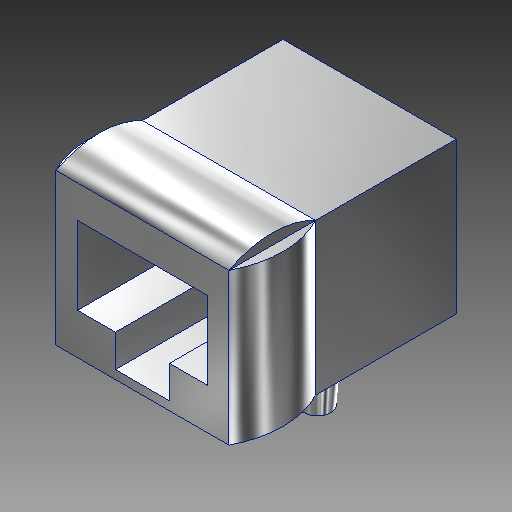
# Autodesk Inventor part: RJ45 Socket
Saved by Autodesk Inventor 2019.4 (Build 234330000, 330)
## iProperties
Created: 2014-11-01
Part Number: RJ45 Socket
Material: Aluminium 6061
Document SubType Name: Modeling
Designer: AndreR
Mass: 10.7449 g
Surface Area: 22.49 cm^2
Volume: 3.96489 cm^3
Density: 2.71 g/cm^3
Appearance: Aluminium - flach
Author: AndreR
Autodesk Inventor part; units mm, degrees
ref_plane "YZ Plane" through (0, 0, 0) normal (1, 0, 0) x (0, 1, 0)
ref_plane "XZ Plane" through (0, 0, 0) normal (0, 1, 0) x (-1, 0, 0)
ref_plane "XY Plane" through (0, 0, 0) normal (0, 0, 1) x (1, 0, 0)
sketch "Skizze1" plane through (0, 0, 0) normal (0, 0, 1) x (1, 0, 0)
  line L0 (-8, 10.5) -> (8, 10.5)
  line L1 (8, 10.5) -> (8, -10.5)
  line L2 (8, -10.5) -> (-8, -10.5)
  line L3 (-8, -10.5) -> (-8, 10.5)
  line L4 (0, 14.7) -> (0, -14.7) projected
  line L5 (-11.2, 0) -> (11.2, 0) projected
  point P0 (0, 0)
  dimension "d0" = 16
  dimension "d2" = 21
  constraints: 8 end point, 2 parallel, 1 horizontal, 1 perpendicular, 2 other
  measures "d0" distance of L0.start L0.end
  measures "d2" distance of L2.end L0.start
extrude "Extrusion1" add sketch "Skizze1" along normal blind 14
sketch "Skizze2" plane through (-8, -10.5, 0) normal (0, -1, 0) x (1, 0, 0)
  line L0 (2, 11) -> (14, 11)
  line L1 (14, 11) -> (14, 3.8)
  line L2 (2, 3.8) -> (2, 11)
  line L3 (10.5, 3.8) -> (10.5, 0.8)
  line L4 (10.5, 0.8) -> (5.5, 0.8)
  line L5 (5.5, 0.8) -> (5.5, 3.8)
  line L6 (16, 0) -> (0, 0) projected
  line L7 (16, 0) -> (16, 14) projected
  line L8 (0, 14) -> (16, 14) projected
  line L9 (0, 0) -> (0, 14) projected
  line L10 (8, 14) -> (8, 0) construction
  line L11 (14, 3.8) -> (10.5, 3.8)
  line L12 (5.5, 3.8) -> (2, 3.8)
  dimension "d5" = 3
  dimension "d6" = 0.8
  dimension "d8" = 2
  dimension "d9" = 5
  dimension "d10" = 3
  constraints: 18 end point, 4 parallel, 2 perpendicular, 1 horizontal, 1 midpoint, 3 other
  measures "d5" distance between parallel lines of L0 L8
  measures "d6" distance between parallel lines of L4 L6
  measures "d8" distance between parallel lines of L1 L7
  measures "d9" distance of L3.end L4.end
  measures "d10" distance between parallel lines of L4 L11
extrude "Extrusion2" cut sketch "Skizze2" against normal blind 10 contours L0 L1 L11 L3 L4 L5 L12 L2
sketch "Skizze3" plane through (0, 0, 0) normal (0, 0, -1) x (-1, 0, 0)
  line L0 (-8, -10.5) -> (8, -10.5) projected
  line L1 (-8, 10.5) -> (-8, -10.5) projected
  line L2 (8, -10.5) -> (8, 10.5) projected
  line L3 (-5.7, 0) -> (5.7, 0) construction
  line L4 (0, -14.7) -> (0, 14.7) construction
  circle A0 centre (-5.7, 0) radius 1.5
  circle A1 centre (5.7, 0) radius 1.5
  point P0 (0, 0)
  dimension "d13" = 10.5
  dimension "d14" = 11.4
  dimension "d15" = 3
  dimension "d16" = 3
  constraints: 2 centre point, 2 coincident, 2 end point, 1 perpendicular, 1 symmetric about line
  measures "d13" distance between parallel lines of L0 L3
  measures "d14" distance of L3.end L3.start
  measures "d15" diameter of A0
  measures "d16" diameter of A1
extrude "Extrusion3" add sketch "Skizze3" along normal blind 3.2 draft -5
sketch "Skizze4" plane through (-8, -10.5, 0) normal (-1, 0, 0) x (0, 0, 1)
  line L0 (14, 21) -> (14, 0) projected
  arc A0 (14, 0) -> (14, 8) centre (6.5, 4) ccw
  line L1 (14, 0) -> (14, 8)
  point P0 (0, 10.5)
  dimension "d19" = 1
  dimension "d20" = 8
  constraints: 2 end point, 2 point on circle, 1 centre point, 1 collinear, 1 point on line
  measures "d19" distance edge to line of A0 L0
  measures "d20" distance of L1.end L0.end
extrude "Extrusion4" add sketch "Skizze4" against normal blind 16
sketch "Skizze5" plane through (0, 0, 14) normal (0, 0, 1) x (1, 0, 0)
  line L0 (-8, 10.5) -> (-8, -10.5) projected
  line L1 (8, -10.5) -> (8, 10.5) projected
  arc A0 (-8, -2.5) -> (-8, -10.5) centre (-0.5, -6.5) ccw
  line L2 (-8, -10.5) -> (-8, -2.5)
  point P0 (0, 0)
  dimension "d23" = 1
  dimension "d24" = 8
  constraints: 2 end point, 2 point on circle, 1 centre point, 1 collinear, 1 point on line
  measures "d23" distance edge to line of A0 L0
  measures "d24" distance of L2.end L0.end
extrude "Extrusion5" add sketch "Skizze5" against normal blind 14
mirror "Spiegeln1" about plane through (0, 0, 0) normal (1, 0, 0) of "Extrusion5"
